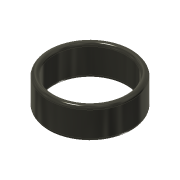
# Autodesk Inventor part: M15 - TX Coil
Saved by Autodesk Inventor 2016 (Build 200138000, 138)
## iProperties
Created: 2017-02-27
Part Number: M15 - TX Coil
Material: SAE 1020
Document SubType Name: Modeling
Designer: Fernando
Stock Number: 0
Mass: 323.712 g
Surface Area: 159.611 cm^2
Volume: 41.1324 cm^3
Density: 7.87 g/cm^3
Appearance: Gunmetal
SurfaceArea_m2: .02
Author: Fernando
Autodesk Inventor part; units mm, degrees
ref_plane "YZ Plane" through (0, 0, 0) normal (1, 0, 0) x (0, 1, 0)
ref_plane "XZ Plane" through (0, 0, 0) normal (0, 1, 0) x (-1, 0, 0)
ref_plane "XY Plane" through (0, 0, 0) normal (0, 0, 1) x (1, 0, 0)
sketch "Sketch2" plane through (0, 0, 0) normal (0, 0, 1) x (1, 0, 0)
  circle A0 centre (0, 0) radius 35
  circle A1 centre (0, 0) radius 41
  dimension "d11" = 6
  dimension "d12" = 70
  constraints: 2 centre point, 2 coincident
  measures "d11" radial gap between concentric circles of A0 A1
  measures "d12" diameter of A0
extrude "Extrusion2" add sketch "Sketch2" along normal blind 30
fillet "Fillet1" radius 3 4 edges at (-35, 0, 30) (-41, 0, 30) (-35, 0, 0) (-41, 0, 0)
body "Solid2"
